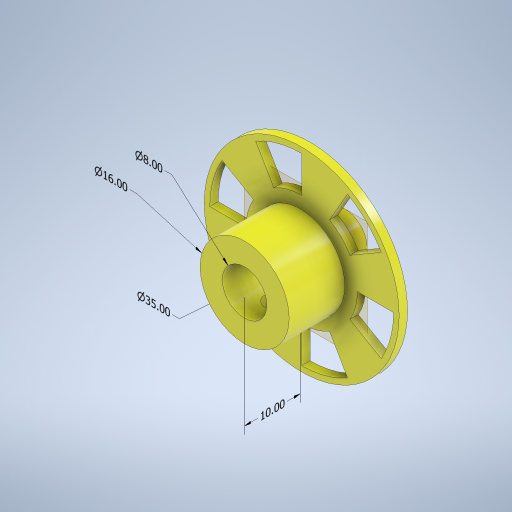
# Autodesk Inventor part: Acople
Saved by Autodesk Inventor 2023 (Build 270158000, 158)
## iProperties
Created: 2022-12-05
Part Number: Acople
Material: Genérico
Document SubType Name: Modeling
Designer: sergi
Density: 1 g/cm^3
Appearance: Valor por defecto
Author: sergi
Autodesk Inventor part; units mm, degrees
ref_plane "YZ Plane" through (0, 0, 0) normal (1, 0, 0) x (0, 1, 0)
ref_plane "XZ Plane" through (0, 0, 0) normal (0, 1, 0) x (-1, 0, 0)
ref_plane "XY Plane" through (0, 0, 0) normal (0, 0, 1) x (1, 0, 0)
sketch "Boceto1" plane through (0, 0, 0) normal (0, 0, 1) x (1, 0, 0)
  circle A0 centre (0, 0) radius 4
  circle A1 centre (0, 0) radius 1.5 projected
  line L0 (0, -1) -> (1.5, -1)
  line L1 (1.5, -1) -> (-2.7531, -1)
  point P0 (1, -1.118)
  point P1 (1, 1.118)
  point P2 (-1.118, -1)
  point P3 (1.118, -1)
  dimension "d0" = 8
  constraints: 4 end point, 1 centre point, 1 coincident, 1 point on line
  measures "d0" diameter of A0
extrude "Extrusión1" add sketch "Boceto1" along normal blind 8 contours A0 | L1 L0 A1 picked at (-0.6553, -1.0791)
sketch "Boceto2" plane through (0, 0, 8) normal (0, 0, 1) x (1, 0, 0)
  circle A0 centre (0, 0) radius 8
  dimension "d3" = 16
  constraints: 1 centre point, 1 coincident
  measures "d3" diameter of A0
extrude "Extrusión2" add sketch "Boceto2" along normal blind 10
sketch "Boceto3" plane through (0, 0, 18) normal (0, 0, 1) x (1, 0, 0)
  circle A0 centre (0, 0) radius 8 projected
  constraints: 1 coincident
hole "Agujero1" at (0, 0, 18) direction (0, 0, -1) diameter 8 depth 8
sketch "Boceto5" plane through (0, 0, 0) normal (0, 1, 0) x (-1, 0, 0)
  line L0 (0, 0) -> (0, 4)
  circle A0 centre (0, 4) radius 1
  line L1 (0, 4) -> (0, 8)
  line L2 (0, 8) -> (0, 13)
  circle A1 centre (0, 13) radius 1.5
  dimension "d20" = 4
  dimension "d21" = 2
  dimension "d29" = 5
  dimension "d30" = 3
  constraints: 6 end point, 2 centre point, 2 coincident, 2 vertical, 1 point on line
  measures "d20" distance of L0.start L0.end
  measures "d21" diameter of A0
  measures "d29" distance of L1.end L2.end
  measures "d30" diameter of A1
hole "Agujero3" at (0, 0, 4) direction (0, -1, 0) diameter 2 end through all
sketch "Boceto6" plane through (0, 0, 0) normal (0, 1, 0) x (-1, 0, 0)
  line L0 (0, 0) -> (0, 13)
  circle A0 centre (0, 13) radius 1.5
  dimension "d31" = 13
  dimension "d32" = 3
  constraints: 2 end point, 1 centre point, 1 coincident, 1 vertical
  measures "d31" distance of L0.start L0.end
  measures "d32" diameter of A0
hole "Agujero4" at (0, 0, 13) direction (0, -1, 0) diameter 3 end through all
ref_plane "Plano de trabajo2" through (0, 0, 7) normal (0, 0, 1) x (-1, 0, 0)
sketch "Boceto7" plane through (0, 0, 7) normal (0, 0, 1) x (-1, 0, 0)
  circle A0 centre (0, 0) radius 17.5
  dimension "d42" = 35
  constraints: 1 centre point, 1 coincident
  measures "d42" diameter of A0
extrude "Extrusión3" add sketch "Boceto7" along normal mid plane 1.5
sketch "Boceto8" plane through (0, 0, 7.75) normal (0, 0, 1) x (1, 0, 0)
  circle A0 centre (0, 0) radius 8 projected
  circle A1 centre (0, 0) radius 17.5 projected
  arc A2 (8.6603, -5) -> (10, 0) centre (0, 0) ccw
  arc A3 (14.2894, -8.25) -> (16.5, 0) centre (0, 0) ccw
  line L0 (10, 0) -> (16.5, 0)
  line L1 (0, 0) -> (16.5, 0) construction
  line L2 (8.6603, -5) -> (14.2894, -8.25)
  arc A4 (8.6603, 5) -> (5, 8.6603) centre (0, 0) ccw
  line L3 (8.6603, 5) -> (14.2894, 8.25)
  arc A5 (14.2894, 8.25) -> (8.25, 14.2894) centre (0, 0) ccw
  line L4 (5, 8.6603) -> (8.25, 14.2894)
  arc A6 (0, 10) -> (-5, 8.6603) centre (0, 0) ccw
  line L5 (0, 10) -> (0, 16.5)
  arc A7 (0, 16.5) -> (-8.25, 14.2894) centre (0, 0) ccw
  line L6 (-5, 8.6603) -> (-8.25, 14.2894)
  arc A8 (-8.6603, 5) -> (-10, 0) centre (0, 0) ccw
  line L7 (-8.6603, 5) -> (-14.2894, 8.25)
  arc A9 (-14.2894, 8.25) -> (-16.5, 0) centre (0, 0) ccw
  line L8 (-10, 0) -> (-16.5, 0)
  arc A10 (-8.6603, -5) -> (-5, -8.6603) centre (0, 0) ccw
  line L9 (-8.6603, -5) -> (-14.2894, -8.25)
  arc A11 (-14.2894, -8.25) -> (-8.25, -14.2894) centre (0, 0) ccw
  line L10 (-5, -8.6603) -> (-8.25, -14.2894)
  arc A12 (0, -10) -> (5, -8.6603) centre (0, 0) ccw
  line L11 (0, -10) -> (0, -16.5)
  arc A13 (0, -16.5) -> (8.25, -14.2894) centre (0, 0) ccw
  line L12 (5, -8.6603) -> (8.25, -14.2894)
  point P0 (0, 0)
  dimension "d45" = 2
  dimension "d46" = 1
  dimension "d50" = 360
  constraints: 26 end point, 24 point on circle, 12 centre point, 2 coincident, 2 horizontal, 1 point on line, 59 other
  measures "d45" radial gap between concentric circles of A0 A2
  measures "d46" radial gap between concentric circles of A1 A3
extrude "Extrusión4" cut sketch "Boceto8" against normal through all contours A2 L0 A3 L2 | A4 L4 A5 L3 | A6 L6 A7 L5 | A8 L8 A9 L7 | A10 L10 A11 L9 | A12 L12 A13 L11
sketch "Boceto9" plane through (0, 0, 0) normal (0, 0, -1) x (-1, 0, 0)
  circle A0 centre (0, 0) radius 1.75
  dimension "d54" = 3.5
  constraints: 1 centre point, 1 coincident
  measures "d54" diameter of A0
extrude "Extrusión5" cut sketch "Boceto9" against normal blind 1.5
sketch "Boceto10" plane through (0, 0, 10) normal (0, 0, 1) x (1, 0, 0)
  arc A0 (1.118, -1) -> (-1.118, -1) centre (0, 0) ccw projected
  circle A1 centre (0, 0) radius 1.75 projected
  line L0 (1.118, -1) -> (-1.118, -1) projected
  point P0 (-1.4361, -1)
  point P1 (-1.7451, -0.1303)
  constraints: 1 other
extrude "Extrusión6" cut sketch "Boceto10" against normal blind 10 contours L0 A0
fillet "Empalme3" radius 2 1 edges at (-4, 0, 6.25)
